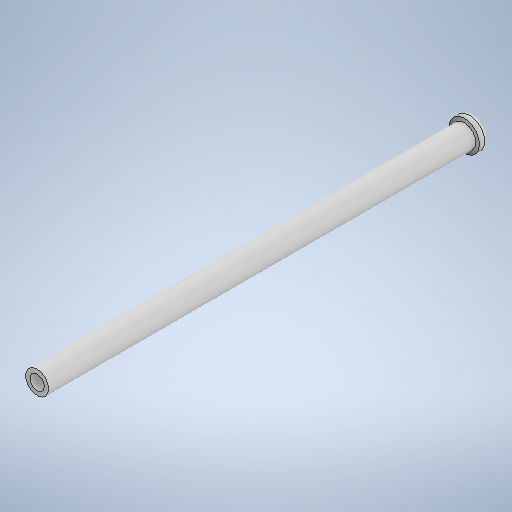
# Autodesk Inventor part: Schanier pin
Saved by Autodesk Inventor 2025.2 (Build 292293000, 293)
## iProperties
Created: 2024-12-16
Part Number: Schanier pin
Material: Generic
Document SubType Name: Modeling
Designer: jurre
Density: 1 g/cm^3
Appearance: Default
Author: jurre
Autodesk Inventor part; units mm, degrees
ref_plane "YZ Plane" through (0, 0, 0) normal (1, 0, 0) x (0, 1, 0)
ref_plane "XZ Plane" through (0, 0, 0) normal (0, 1, 0) x (-1, 0, 0)
ref_plane "XY Plane" through (0, 0, 0) normal (0, 0, 1) x (1, 0, 0)
sketch "Sketch1" plane through (0, 0, 0) normal (0, 0, 1) x (1, 0, 0)
  circle A0 centre (0, 0) radius 2.175
  circle A1 centre (0, 0) radius 1.75
  circle A2 centre (0, 0) radius 2.875
  circle A3 centre (0, 0) radius 2.25
  dimension "d0" = 4.35
  dimension "d1" = 3.5
  dimension "d2" = 5.75
  dimension "d3" = 4.5
  constraints: 4 centre point, 4 coincident
  measures "d0" diameter of A0
  measures "d1" diameter of A1
  measures "d2" diameter of A2
  measures "d3" diameter of A3
extrude "Extrusion1" add sketch "Sketch1" along normal blind 81 contours A0 | A1
extrude "Extrusion2" add sketch "Sketch1" against normal blind 2 contours A0 | A1 | A2 | A3
fillet "Fillet1" radius 1 1 edges at (-2.875, 0, -2)
sketch "Sketch2" plane through (0, 0, 81) normal (0, 0, 1) x (1, 0, 0)
  circle A0 centre (0, 0) radius 1.375
  dimension "d9" = 2.75
  constraints: 1 centre point, 1 coincident
  measures "d9" diameter of A0
extrude "Extrusion3" cut sketch "Sketch2" against normal blind 6
body "Solid1"
